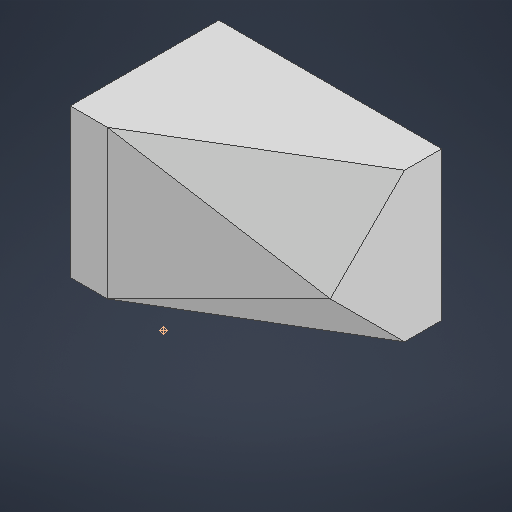
# Autodesk Inventor part: B6
Saved by Autodesk Inventor 2025.4 (Build 294407000, 407)
## iProperties
Created: 2026-05-14
Part Number: B6
Material: Generic
Document SubType Name: Modeling
Designer: VuQuan
Density: 1 g/cm^3
Appearance: Default
Author: VuQuan
Autodesk Inventor part; units mm, degrees
ref_plane "YZ Plane" through (0, 0, 0) normal (1, 0, 0) x (0, 1, 0)
ref_plane "XZ Plane" through (0, 0, 0) normal (0, 1, 0) x (-1, 0, 0)
ref_plane "XY Plane" through (0, 0, 0) normal (0, 0, 1) x (1, 0, 0)
sketch "Sketch1" plane through (0, 0, 0) normal (0, 0, 1) x (1, 0, 0)
  line L0 (-5, 40) -> (55, 40)
  line L1 (55, 40) -> (55, 10)
  line L2 (5, 0) -> (-5, 0)
  line L3 (-5, 0) -> (-5, 40)
  line L4 (55, 10) -> (5, 0)
  point P0 (0, 0)
  point P1 (55, 0)
  point P2 (0, 0)
  dimension "d0" = 40
  dimension "d1" = 60
  dimension "d2" = 10
  dimension "d3" = 50
  constraints: 10 end point, 2 parallel, 2 point on line, 1 coincident, 1 horizontal, 1 midpoint, 1 perpendicular
  measures "d0" distance of L0.end point (55, 0)
  measures "d1" distance of point (55, 0) L2.end
  measures "d2" distance of L1.end point (55, 0)
  measures "d3" distance of L2.start point (55, 0)
extrude "Extrusion1" add sketch "Sketch1" against normal blind 40
sketch "Sketch2" plane through (55, 10, 0) normal (1, 0, 0) x (0, 0, -1)
  line L0 (0, 0) -> (0, 30) projected
  line L1 (0, 0) -> (40, 0) projected
  line L2 (40, 30) -> (40, 0) projected
  line L3 (20, 0) -> (0, 20)
  line L4 (20, 0) -> (40, 20)
  point P0 (0, -10)
  dimension "d6" = 20
  constraints: 4 end point, 2 midpoint, 2 point on line, 1 horizontal alignment
  measures "d6" horizontal distance of L3.end point (20, 0)
sketch "Sketch3" plane through (0, 0, 0) normal (0, 0, 1) x (1, 0, 0)
  line L0 (5, 0) -> (55, 30)
  line L1 (55, 10) -> (55, 30) projected
  point P0 (0, 0)
  constraints: 2 end point
sweep "Sweep1" cut profiles "Sketch2" path "Sketch3" path curves L0
move or copy body "Rotate1" bodies to move or copy 1 copy no rotation origin (0, 0, 0) rotation axis (1, 0, 0) rotation angle -90 translate (0, 60, 20)
body "Solid1"
